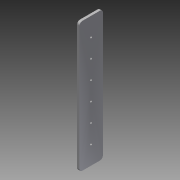
# Autodesk Inventor part: joinerBracket
Saved by Autodesk Inventor 2014 (Build 180170000, 170)
## iProperties
Created: 2014-09-15
Part Number: joinerBracket
Material: Steel
Document SubType Name: Modeling
Designer: Dave
Mass: 115.602 g
Surface Area: 125.495 cm^2
Volume: 14.7264 cm^3
Density: 7.85 g/cm^3
Appearance: Steel
Author: Dave
Autodesk Inventor part; units mm, degrees
ref_plane "YZ Plane" through (0, 0, 0) normal (1, 0, 0) x (0, 1, 0)
ref_plane "XZ Plane" through (0, 0, 0) normal (0, 1, 0) x (-1, 0, 0)
ref_plane "XY Plane" through (0, 0, 0) normal (0, 0, 1) x (1, 0, 0)
sketch "Sketch1" plane through (0, 0, 0) normal (1, 0, 0) x (0, 1, 0)
  line L0 (3.175, 0) -> (136.825, 0)
  line L1 (140, -3.175) -> (140, -22.225)
  line L2 (136.825, -25.4) -> (3.175, -25.4)
  line L3 (0, -22.225) -> (0, -3.175)
  arc A0 (140, -3.175) -> (136.825, 0) centre (136.825, -3.175) ccw
  arc A1 (136.825, -25.4) -> (140, -22.225) centre (136.825, -22.225) ccw
  arc A2 (0, -22.225) -> (3.175, -25.4) centre (3.175, -22.225) ccw
  arc A3 (3.175, 0) -> (0, -3.175) centre (3.175, -3.175) ccw
  point P0 (0, 0)
  point P1 (140, 0)
  point P2 (0, -25.4)
  dimension "d0" = 25.4
  dimension "d1" = 140
  dimension "d2" = 3.175
  constraints: 8 end point, 8 point on circle, 8 tangent, 6 point on line, 4 centre point, 3 equal radius, 2 parallel, 1 horizontal, 1 perpendicular
  measures "d0" distance of point (0, -25.4) point (0, 0)
  measures "d1" distance of point (0, 0) point (140, 0)
  measures "d2" radius of A0
extrude "Extrusion1" add sketch "Sketch1" along normal blind 2.54
sketch "Sketch3" plane through (2.54, 0, 0) normal (1, 0, 0) x (0, 0, -1)
  line L0 (22.225, 140) -> (3.175, 140) projected
  line L1 (0, 136.825) -> (0, 3.175) projected
  circle A0 centre (12.7, 120) radius 1.9226
  circle A1 centre (12.7, 100) radius 1.9226
  circle A2 centre (12.7, 80) radius 1.9226
  circle A3 centre (12.7, 60) radius 1.9226
  circle A4 centre (12.7, 40) radius 1.9226
  circle A5 centre (12.7, 20) radius 1.9226
  point P0 (0, 0)
  dimension "d29" = 20
  dimension "d32" = 20
  constraints: 6 centre point, 1 vertical, 10 other
  measures "d29" distance from line of A0.centre L0
  measures "d32" distance of A0.centre A1.centre
hole "Hole2" at (2.54, 40, -12.7) at (2.54, 20, -12.7) at (2.54, 60, -12.7) at (2.54, 80, -12.7) at (2.54, 100, -12.7) at (2.54, 120, -12.7) direction (-1, 0, 0) diameter 2 depth 25.4 tip angle 118
body "Solid1"
